speaker_mount (Autodesk Fusion 360 design; units mm, degrees)
Autodesk Fusion 360 part; units mm, degrees
sketch "Sketch1" plane through (0, 0, 0) normal (0, 0, 1) x (1, 0, 0)
  line L0 (54.7723, 15) -> (57, 15)
  line L1 (60, 12) -> (60, -12)
  line L2 (57, -15) -> (54.7723, -15)
  line L3 (-60, -12) -> (-60, 12)
  line L4 (0, 0) -> (-72.9776, 0) construction
  arc A0 (12.5996, -30.5) -> (-12.5996, -30.5) centre (0, 0) ccw
  arc A1 (-22.5533, -26.7647) -> (-19.681, -28.9423) centre (0, 0) ccw
  arc A2 (19.681, -28.9423) -> (22.5533, -26.7647) centre (0, 0) ccw
  line L5 (-57, 15) -> (-54.7723, 15)
  line L6 (-57, -15) -> (-54.7723, -15)
  arc A3 (22.5533, 26.7647) -> (54.7723, 15) centre (54.7723, 65) ccw
  arc A4 (-54.7723, 15) -> (-22.5533, 26.7647) centre (-54.7723, 65) ccw
  arc A5 (54.7723, -15) -> (22.5533, -26.7647) centre (54.7723, -65) ccw
  arc A6 (-22.5533, -26.7647) -> (-54.7723, -15) centre (-54.7723, -65) ccw
  arc A7 (-57, 15) -> (-60, 12) centre (-57, 12) ccw
  arc A8 (-60, -12) -> (-57, -15) centre (-57, -12) ccw
  arc A9 (60, 12) -> (57, 15) centre (57, 12) ccw
  arc A10 (57, -15) -> (60, -12) centre (57, -12) ccw
  arc A11 (11.3617, -28.3048) -> (-11.3617, -28.3048) centre (0, 0) ccw
  circle A12 centre (-50, 0) radius 2.25
  line L7 (60, 0) -> (50, 0) construction
  circle A13 centre (50, 0) radius 2.25
  circle A14 centre (0, 0) radius 30.5
  circle A15 centre (0, 0) radius 33
  arc A16 (-22.5533, -26.7647) -> (-12.1795, -32.8125) centre (0, 0) ccw
  arc A17 (12.1795, -32.8125) -> (22.5533, -26.7647) centre (0, 0) ccw
  arc A18 (11.1355, -33) -> (12.1795, -32.8125) centre (11.1355, -30) ccw
  arc A19 (-12.1795, -32.8125) -> (-11.1355, -33) centre (-11.1355, -30) ccw
  line L8 (8.3066, 34) -> (-8.3066, 34)
  line L9 (-7.5498, -34) -> (7, -34)
  line L10 (7, -34) -> (7.5498, -34)
  arc A20 (-11.1355, -33) -> (-7.5498, -34) centre (0, 0) ccw
  arc A21 (7.5498, -34) -> (11.1355, -33) centre (0, 0) ccw
  arc A22 (22.5533, 26.7647) -> (8.3066, 34) centre (0, 0) ccw
  arc A23 (-8.3066, 34) -> (-22.5533, 26.7647) centre (0, 0) ccw
  arc A24 (22.5533, 26.7647) -> (8.3066, 34) centre (0, 0) ccw
  arc A25 (-8.3066, 34) -> (-22.5533, 26.7647) centre (0, 0) ccw
  point P0 (-60, 15)
  point P1 (60, 15)
  point P2 (-60, -15)
  point P3 (-60, 0)
  point P4 (0, -33)
  point P5 (0, 33)
  dimension "d1" = 61
  dimension "d2" = 66
  dimension "d3" = 70
  dimension "d4" = 30
  dimension "d5" = 120
  dimension "d6" = 50
  dimension "d7" = 50
  dimension "d8" = 50
  dimension "d9" = 50
  dimension "d10" = 3
  dimension "d11" = 3
  dimension "d12" = 3
  dimension "d13" = 3
  dimension "d20" = 4.5
  dimension "d21" = 10
  dimension "d22" = 4.5
  dimension "d23" = 10
  dimension "d28" = 3
  dimension "d30" = 1
  dimension "d31" = 1
  constraint coincident L4.start A0.centre
  constraint concentric A0 A2
  constraint horizontal L0
  constraint vertical L1
  constraint horizontal L2
  constraint vertical L3
  constraint perpendicular L3 L4
  constraint coincident P3 L4
  constraint concentric A1 A2
  constraint concentric A2 A22
  constraint tangent A3 A22
  constraint tangent L0 A3
  constraint tangent L5 A4
  constraint tangent A4 A22
  constraint tangent L2 A5
  constraint tangent A2 A5
  constraint tangent L6 A6
  constraint tangent A1 A6
  constraint coincident L3 P3
  constraint coincident P0 L5
  constraint coincident P0 L3
  constraint tangent L5 A7
  constraint tangent L3 A7
  constraint coincident P2 L3
  constraint coincident P2 L6
  constraint tangent L3 A8
  constraint tangent L6 A8
  constraint coincident P1 L0
  constraint coincident P1 L1
  constraint tangent L0 A9
  constraint tangent L1 A9
  constraint tangent L1 A10
  constraint tangent L2 A10
  constraint coincident L4 A12.centre
  constraint midpoint L1 L7.start
  constraint perpendicular L1 L7
  constraint coincident L7.end A13.centre
  constraint concentric A0 A14
  constraint concentric A2 A15
  constraint concentric A17 A22
  constraint concentric A16 A17
  constraint concentric A17 A24
  constraint tangent A17 A18
  constraint tangent A16 A19
  constraint equal A18 A19
  constraint coincident A15 P4
  constraint horizontal L8
  constraint coincident L8.end A24
  constraint midpoint A0 P5
  constraint horizontal L9
  constraint coincident L10.end A20
  constraint parallel L9 L10
  constraint concentric A20 A21
  constraint concentric A22 A23
  constraint concentric A24 A25
  measures "d1" diameter of A11
  measures "d2" diameter of A0
  measures "d3" diameter of A2
  measures "d4" distance of P0 P2
  measures "d5" distance of P0 P1
  measures "d6" radius of A3
  measures "d7" radius of A4
  measures "d8" radius of A5
  measures "d9" radius of A6
  measures "d10" radius of A7
  measures "d11" radius of A8
  measures "d12" radius of A9
  measures "d13" radius of A10
  measures "d20" diameter of A12
  measures "d21" distance of L7.start L7.end
  measures "d22" diameter of A13
  measures "d23" distance of P3 A12.centre
  measures "d28" radius of A18
  measures "d30" distance of L8 P5
  measures "d31" distance of P4 L9
extrude "Extrude1" add sketch "Sketch1" along normal blind 5.5 contours L0 L1 L2 L3 A1 A2 L5 L6 A3 A4 A5 A6 A7 A8 A9 A10 A16 A17 A18 A19 L8 L9 L10 A20 A21 A22 A23 A24 A25
extrude "Extrude2" add sketch "Sketch1" along normal blind 1 contours A0 A15 | A11 A14
extrude "Extrude3" cut sketch "Sketch1" along normal through all contours A11 A14
